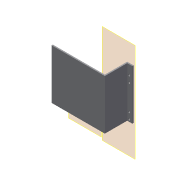
# Autodesk Inventor part: 30_CUBE_openSIM_Lasershield
Saved by Autodesk Inventor 2019 (Build 230136000, 136)
## iProperties
Created: 2020-03-02
Part Number: 30_CUBE_openSIM_Lasershield
Material: Generic
Document SubType Name: Modeling
Designer: diederichbenedict
Density: 1 g/cm^3
Appearance: Default
Author: diederichbenedict
Autodesk Inventor part; units mm, degrees
ref_plane "YZ Plane" through (0, 0, 0) normal (1, 0, 0) x (0, 1, 0)
ref_plane "XZ Plane" through (0, 0, 0) normal (0, 1, 0) x (-1, 0, 0)
ref_plane "Work Plane1" through (0, 0, 0) normal (0, 0, 1) x (1, 0, 0)
ref_plane "Work Plane2" through (0, 0, 0) normal (0, 0, 1) x (1, 0, 0)
sketch "Sketch2" plane through (0, 0, 0) normal (0, 0, 1) x (1, 0, 0)
  circle A0 centre (44.9, -55.1) radius 1.6 construction
  circle A1 centre (44.9, -45.1) radius 1.6 construction
  line L0 (49.9, -97.9) -> (49.9, 41.0746) construction
  line L1 (-49.9, -35.1) -> (-49.9, -97.9) construction
  circle A2 centre (-45.1, -45.1) radius 1.6 construction
  circle A3 centre (-45.1, -55.1) radius 1.4 construction
  line L2 (-2.8791, -35.1) -> (-48.921, -35.1) construction
  circle A4 centre (44.9, -5.1) radius 1.6 construction
  circle A5 centre (44.9, 4.9) radius 1.6 construction
  line L3 (49.9, -58.5557) -> (41.9, -58.5557) construction
  line L4 (41.9, -58.5557) -> (41.9, 19.8666) construction
  line L5 (41.9, 19.8666) -> (49.9, 19.8666) construction
  line L6 (49.9, 19.8666) -> (49.9, -58.5557) construction
  line L7 (41.9, -58.5557) -> (49.9, -58.5557)
  line L8 (49.9, -58.5557) -> (49.9, 19.8666)
  line L9 (49.9, 19.8666) -> (41.9, 19.8666)
  line L10 (41.9, 19.8666) -> (41.9, -58.5557)
  line L11 (41.9, 19.8666) -> (49.9, 36.639)
  line L12 (49.9, 19.8666) -> (49.9, 36.639)
  line L13 (60.4304, 64.9211) -> (17.3793, -25.3374) projected
  line L14 (-49.9, -58.0504) -> (-41.9, -58.0504)
  line L15 (-41.9, -58.0504) -> (-41.9, -38.0504)
  line L16 (-41.9, -38.0504) -> (-49.9, -38.0504)
  line L17 (-49.9, -38.0504) -> (-49.9, -58.0504)
  line L18 (-41.9, -58.0504) -> (-39.9, -58.0504)
  line L19 (-39.9, -58.0504) -> (-39.9, -38.0504)
  line L20 (-39.9, -38.0504) -> (-41.9, -38.0504)
  line L21 (-41.9, -38.0504) -> (-41.9, -58.0504)
  line L22 (41.9, -58.5557) -> (39.9, -58.5557)
  line L23 (39.9, -58.5557) -> (39.9, 19.7918)
  line L24 (39.9, 19.7918) -> (41.9, 19.7918)
  line L25 (41.9, 19.7918) -> (41.9, -58.5557)
  circle A6 centre (-45.1, -55.1) radius 1.4
  circle A7 centre (-45.1, -45.1) radius 1.6
  circle A8 centre (44.9, -55.1) radius 1.6
  circle A9 centre (44.9, -45.1) radius 1.6
  circle A10 centre (44.9, -5.1) radius 1.6
  circle A11 centre (44.9, 4.9) radius 1.6
  line L26 (39.9, -58.5557) -> (9.9, -58.5557)
  line L27 (9.9, -58.5557) -> (9.9, -56.5557)
  line L28 (9.9, -56.5557) -> (39.9, -56.5557)
  line L29 (39.9, -56.5557) -> (39.9, -58.5557)
  point P0 (0, 0)
  dimension "d0" = 8
  dimension "d1" = 8
  dimension "d2" = 20
  dimension "d3" = 2
  dimension "d4" = 2
  dimension "d7" = 30
  dimension "d8" = 2
  constraints: 52 end point, 13 parallel, 6 centre point, 6 coincident, 6 concentric, 6 horizontal, 6 perpendicular, 4 point on line, 1 collinear
  measures "d0" distance of L4.end L5.end
  measures "d1" distance of L16.end L15.end
  measures "d2" distance of L15.end L14.end
  measures "d3" distance of L20.end L19.end
  measures "d4" distance of L23.end L24.end
  measures "d7" distance of L27.end L28.end
  measures "d8" distance of L26.end L27.end
extrude "Extrusion1" add sketch "Sketch2" along normal blind 2 contours L10 L9 L8 L7 | L22 L23 L24 L10 | L26 L27 L28 L23 | L17 L16 L15 L14 | L15 L20 L19 L18
sketch "Sketch3" plane through (0, 0, 2) normal (0, 0, 1) x (1, 0, 0)
  line L0 (39.9, 19.7918) -> (39.9, -56.5557) projected
  circle A0 centre (44.9, 4.9) radius 1.6 projected
  circle A1 centre (44.9, -5.1) radius 1.6 projected
  circle A2 centre (44.9, -45.1) radius 1.6 projected
  circle A3 centre (44.9, -55.1) radius 1.6 projected
  line L1 (39.9, -56.5557) -> (9.9, -56.5557) projected
  line L2 (9.9, -56.5557) -> (9.9, -58.5557) projected
  line L3 (9.9, -58.5557) -> (49.9, -58.5557) projected
  line L4 (49.9, -58.5557) -> (49.9, 19.8666) projected
  line L5 (49.9, 19.8666) -> (41.9, 19.8666) projected
  line L6 (41.9, 19.8666) -> (41.9, 19.7918) projected
  line L7 (41.9, 19.7918) -> (39.9, 19.7918) projected
  line L8 (39.9, 19.7918) -> (39.9, -56.5557) projected
  line L9 (39.9, 19.7918) -> (39.9, -56.5557) projected
  line L10 (9.9, -58.5557) -> (49.9, -58.5557) projected
  line L11 (39.9, 19.7918) -> (41.9, 19.7918)
  line L12 (41.9, 19.7918) -> (41.9, -58.5557)
  line L13 (41.9, -58.5557) -> (39.9, -58.5557)
  line L14 (39.9, -58.5557) -> (39.9, 19.7918)
  line L15 (39.9, -56.5557) -> (9.9, -56.5557) projected
  line L16 (9.9, -58.5557) -> (39.9, -58.5557)
  line L17 (39.9, -58.5557) -> (39.9, -56.5557)
  line L18 (39.9, -56.5557) -> (9.9, -56.5557)
  line L19 (9.9, -56.5557) -> (9.9, -58.5557)
  line L20 (-39.9, -58.0504) -> (-39.9, -38.0504) projected
  line L21 (-49.9, -58.0504) -> (-39.9, -58.0504) projected
  line L22 (-39.9, -38.0504) -> (-41.9, -38.0504)
  line L23 (-41.9, -38.0504) -> (-41.9, -58.0504)
  line L24 (-41.9, -58.0504) -> (-39.9, -58.0504)
  line L25 (-39.9, -58.0504) -> (-39.9, -38.0504)
  point P0 (0, 0)
  dimension "d9" = 2
  constraints: 24 end point, 6 parallel, 3 horizontal, 3 perpendicular, 2 point on line
  measures "d9" distance of L24.end L23.end
ref_plane "Work Plane3" through (-48.921, -35.1, 35.161) normal (0, 0, 1) x (1, 0, 0)
extrude "Extrusion2" add sketch "Sketch3" along normal up to surface (33.161 mm away) contours L7 L12 L3 L14 L0 | L14 L3 L2 L1 | L21 L23 L22 L20
sketch "Sketch5" plane through (9.9, -58.5557, 35.161) normal (0, 0, 1) x (1, 0, 0)
  line L0 (0, 0) -> (0, 2) projected
  line L1 (32, 0) -> (0, 0) projected
  line L2 (32, 78.3475) -> (32, 0) projected
  line L3 (30, 78.3475) -> (32, 78.3475) projected
  line L4 (30, 2) -> (30, 78.3475) projected
  line L5 (0, 2) -> (30, 2) projected
  line L6 (-49.8, 20.5053) -> (-49.8, 0.5053) projected
  line L7 (-51.8, 20.5053) -> (-49.8, 20.5053) projected
  line L8 (-51.8, 0.5053) -> (-51.8, 20.5053) projected
  line L9 (-49.8, 0.5053) -> (-51.8, 0.5053) projected
  line L10 (32, 78.3475) -> (-51.8, 78.3475)
  line L11 (-51.8, 78.3475) -> (-51.8, 0.5053)
  line L12 (-51.8, 0.5053) -> (32, 0.5053)
  line L13 (32, 0.5053) -> (32, 78.3475)
  line L14 (32, 78.3475) -> (32, 0) projected
  line L15 (32, 0) -> (-51.8, 0)
  line L16 (-51.8, 0) -> (-51.8, 0.5053)
  line L17 (-51.8, 0.5053) -> (32, 0.5053)
  line L18 (32, 0.5053) -> (32, 0)
  point P0 (-9.9, 58.5557)
  constraints: 16 end point, 4 parallel, 2 horizontal, 2 perpendicular
extrude "Extrusion3" add sketch "Sketch5" along normal blind 2
sketch "Sketch6" plane through (-41.9, -58.0504, 2) normal (-1, 0, 0) x (0, 0, 1)
  line L0 (0, 20) -> (33.161, 20) projected
  line L1 (0, 0) -> (0, 20) projected
  line L2 (0, 0) -> (33.161, 0) projected
  line L3 (33.161, 0) -> (33.161, -0.5053) projected
  line L4 (33.161, -0.5053) -> (35.161, -0.5053) projected
  line L5 (35.161, 77.8423) -> (35.161, -0.5053) projected
  line L6 (33.161, 77.8423) -> (35.161, 77.8423) projected
  line L7 (33.161, 77.8423) -> (33.161, 20) projected
  line L8 (-2, 7.7504) -> (-2, -86.2156) projected
  line L9 (-2, -86.2156) -> (3, -86.2156) projected
  line L10 (3, -19.7496) -> (3, -86.2156) projected
  line L11 (3, -19.7496) -> (7.1792, -19.7496) projected
  line L12 (7.1792, -19.7496) -> (7.1792, -14.7496) projected
  line L13 (3, -14.7496) -> (7.1792, -14.7496) projected
  line L14 (3, 7.7504) -> (3, -14.7496) projected
  line L15 (-2, 7.7504) -> (3, 7.7504) projected
  line L16 (-2.5429, 8.2795) -> (3.9802, 8.2795)
  line L17 (3.9802, 8.2795) -> (3.9802, -0.9887)
  line L18 (3.9802, -0.9887) -> (-2.5429, -0.9887)
  line L19 (-2.5429, -0.9887) -> (-2.5429, 8.2795)
  point P0 (-2, 58.0504)
  constraints: 8 end point, 2 parallel, 1 horizontal, 1 perpendicular
extrude "Extrusion4" cut sketch "Sketch6" along normal mid plane 20 contours L16 L17 L2 L14 L15 L1 | L1 L15 L8 L18 L19 L16 | L15 L14 L2 L1 | L1 L2 L14 L18 L8 L15 | L17 L18 L14 L2
body "Solid1"
